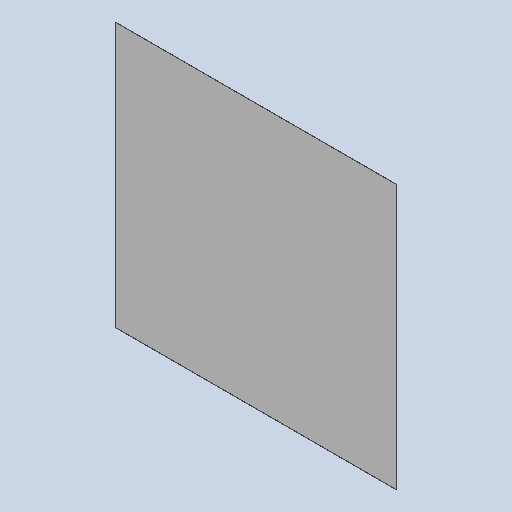
# Autodesk Inventor part: OLED_1_3_CARRIERBOARD-Footprint-1_CMP-00028-00008-2
Saved by Autodesk Inventor 2024.3 (Build 283343000, 343)
## iProperties
Created: 2024-05-05
Part Number: OLED_1_3_CARRIERBOARD-Footprint-1_CMP-00028-00008-2
Material: Generic
Document SubType Name: Modeling
Designer: atrus
Density: 1 g/cm^3
Appearance: Default
Author: atrus
Autodesk Inventor part; units mm, degrees
ref_plane "YZ Plane" through (0, 0, 0) normal (1, 0, 0) x (0, 1, 0)
ref_plane "XZ Plane" through (0, 0, 0) normal (0, 1, 0) x (-1, 0, 0)
ref_plane "XY Plane" through (0, 0, 0) normal (0, 0, 1) x (1, 0, 0)
sketch "Sketch1" plane through (0, 0, 0) normal (0, 0, 1) x (1, 0, 0)
  line L0 (-14.015, -32.076) -> (21.635, -32.076)
  line L1 (21.635, -32.076) -> (21.635, 1.524)
  line L2 (21.635, 1.524) -> (-14.015, 1.524)
  line L3 (-14.015, 1.524) -> (-14.015, -32.076)
  constraints: 8 end point
extrude "Extrusion1" add sketch "Sketch1" along normal blind 0.0254
body "Solid1"
